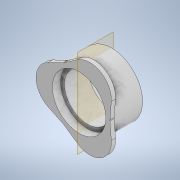
# Autodesk Inventor part: EDF Mount
Saved by Autodesk Inventor 2020 (Build 240168000, 168)
## iProperties
Created: 2020-03-02
Part Number: EDF Mount
Material: Generic
Document SubType Name: Modeling
Designer: pp445
Density: 1 g/cm^3
Appearance: Default
Author: pp445
Autodesk Inventor part; units mm, degrees
ref_plane "XZ Plane" through (0, 0, 0) normal (0, 1, 0) x (-1, 0, 0)
ref_plane "XY Plane" through (0, 0, 0) normal (0, 0, 1) x (1, 0, 0)
sketch "Sketch1" plane through (0, 0, 0) normal (0, 0, 1) x (1, 0, 0)
  circle A0 centre (0, 0) radius 27.575
  circle A1 centre (0, 0) radius 51.5
  dimension "d0" = 55.15
  dimension "d1" = 103
  constraints: 2 centre point, 2 coincident
  measures "d0" diameter of A0
  measures "d1" diameter of A1
extrude "Extrusion1" add sketch "Sketch1" along normal blind 39
sketch "Sketch2" plane through (0, 0, 0) normal (1, 0, 0) x (0, 1, 0)
  line L0 (51.5, 39) -> (-51.5, 39) projected
  line L1 (51.5, 0) -> (-51.5, 0) projected
  line L2 (42.7787, 29) -> (-54.5799, 29) construction
  line L3 (-27.575, 39) -> (27.575, 39) projected
  line L4 (-27.575, 39) -> (27.575, 39) projected
  line L5 (-27.575, 0) -> (27.575, 0) projected
  line L6 (51.5, 0) -> (27.575, 0) projected
  line L7 (27.575, 0) -> (27.575, 39) projected
  line L8 (27.575, 39) -> (51.5, 39) projected
  line L9 (-51.5, 39) -> (-27.575, 39) projected
  line L10 (-27.575, 39) -> (-27.575, 0) projected
  line L11 (-27.575, 0) -> (-51.5, 0) projected
  line L12 (27.575, 39) -> (32, 39)
  line L13 (32, 39) -> (32, 29)
  line L14 (32, 29) -> (27.575, 29)
  line L15 (27.575, 29) -> (27.575, 39)
  line L16 (0, -7.8) -> (0, 46.8) projected
  line L17 (51.5, 39) -> (51.5, 0) projected
  line L18 (-51.5, 0) -> (-51.5, 39) projected
  point P0 (0, 0)
  dimension "d4" = 10
  dimension "d5" = 32
  constraints: 10 end point, 3 parallel, 1 collinear, 1 horizontal, 1 perpendicular
  measures "d4" distance between parallel lines of L0 L2
  measures "d5" distance from line of point (0, 0) L13
revolve "Revolution1" cut sketch "Sketch2" angle 360 about axis through (0, 0, -10) along (0, 0, 1) contours L13 L14 L7 L0
sketch "Sketch3" plane through (0, 0, 0) normal (1, 0, 0) x (0, 1, 0)
  line L0 (51.5, 39) -> (51.5, 0) projected
  line L1 (51.5, 0) -> (27.575, 0) projected
  line L2 (27.575, 0) -> (27.575, 29) projected
  line L3 (27.575, 29) -> (32, 29) projected
  line L4 (32, 29) -> (32, 39) projected
  line L5 (32, 39) -> (51.5, 39) projected
  line L6 (-51.5, 0) -> (-51.5, 39) projected
  line L7 (-51.5, 39) -> (-32, 39) projected
  line L8 (-32, 39) -> (-32, 29) projected
  line L9 (-32, 29) -> (-27.575, 29) projected
  line L10 (-27.575, 29) -> (-27.575, 0) projected
  line L11 (-27.575, 0) -> (-51.5, 0) projected
  line L12 (-51.5, 0) -> (-51.5, 39) projected
  line L13 (-32, 39) -> (-32, 29) projected
  line L14 (-32, 34) -> (-51.5, 34)
  line L15 (-37, 34) -> (-37, 0)
  line L16 (51.5, 0) -> (-51.5, 0) projected
  line L17 (0, -7.8) -> (0, 46.8) projected
  point P0 (0, 0)
  point P1 (-51.5, 34)
  dimension "d7" = 5
  dimension "d11" = 5
  constraints: 4 end point, 3 point on line, 1 midpoint, 1 parallel, 1 perpendicular
  measures "d7" distance between parallel lines of L7 L14
  measures "d11" distance between parallel lines of L8 L15
revolve "Revolution2" cut sketch "Sketch3" angle 360 about axis through (0, 0, -10) along (0, 0, 1) contours L6 L14 L15 L11
sketch "Sketch4" plane through (0, 0, 39) normal (0, 0, 1) x (1, 0, 0)
  circle A0 centre (0, 0) radius 32 projected
  circle A1 centre (0, 0) radius 51.5 projected
  circle A2 centre (0, 0) radius 32 projected
  line L0 (0, 0) -> (-55.0177, 0) construction
  line L1 (0, 0) -> (34.9883, -60.6016) construction
  line L2 (0, 0) -> (42.9469, 74.3862) construction
  circle A3 centre (-25.75, 0) radius 25.75 construction
  circle A4 centre (12.875, -22.3002) radius 25.75 construction
  circle A5 centre (0, 0) radius 51.5 projected
  circle A6 centre (12.875, 22.3002) radius 25.75 construction
  line L3 (0, 0) -> (-33.8932, -58.7048) construction
  line L4 (0, 0) -> (-35.029, 60.6721) construction
  line L5 (0, 0) -> (41.9391, 0) construction
  circle A7 centre (-22.125, -38.3216) radius 7.25 construction
  circle A8 centre (-22.125, 38.3216) radius 7.25 construction
  circle A9 centre (44.25, 0) radius 7.25 construction
  line L6 (38.5484, -20.3161) -> (37.0216, -0.5586)
  line L7 (38.5484, 20.3161) -> (37.0216, 0.5586)
  line L8 (-1.68, -43.542) -> (-18.027, -32.3409)
  line L9 (-36.8684, -23.2259) -> (-18.9946, -31.7823)
  line L10 (-36.8684, 23.2259) -> (-18.9946, 31.7823)
  line L11 (-18.027, 32.3409) -> (-1.68, 43.542)
  arc A10 (-1.68, -43.542) -> (38.5484, -20.3161) centre (12.875, -22.3002) ccw
  arc A11 (37.0216, 0.5586) -> (37.0216, -0.5586) centre (44.25, 0) ccw
  arc A12 (36.3356, 11.6859) -> (-1.68, 43.542) centre (12.875, 22.3002) ccw
  arc A13 (-18.9946, 31.7823) -> (-18.027, 32.3409) centre (-22.125, 38.3216) ccw
  arc A14 (-18.027, -32.3409) -> (-18.9946, -31.7823) centre (-22.125, -38.3216) ccw
  arc A15 (-36.8684, 23.2259) -> (-36.8684, -23.2259) centre (-25.75, 0) ccw
  circle A16 centre (0, 0) radius 37 projected
  point P0 (-51.5, 0)
  point P1 (25.75, -44.6003)
  point P2 (25.75, 44.6003)
  dimension "d12" = 120
  dimension "d13" = 120
  dimension "d14" = 120
  dimension "d15" = 120
  constraints: 28 point on circle, 24 end point, 22 tangent, 12 centre point, 7 point on line, 5 coincident, 2 horizontal
  measures "d12" angle of L0 L1
  measures "d13" angle of L2 L1
  measures "d14" angle of L5 L3
  measures "d15" angle of L3 L4
extrude "Extrusion2" cut sketch "Sketch4" against normal up to surface (5 mm away) contours A1 A10 L6 A11 L7 A12 | A12 L11 A13 L10 A15 A1 | A1 A15 L9 A14 L8 A10
equation "\"d13\" = d12"
equation "\"d14\" = d12"
equation "\"d15\" = d12"
body "Solid1"
